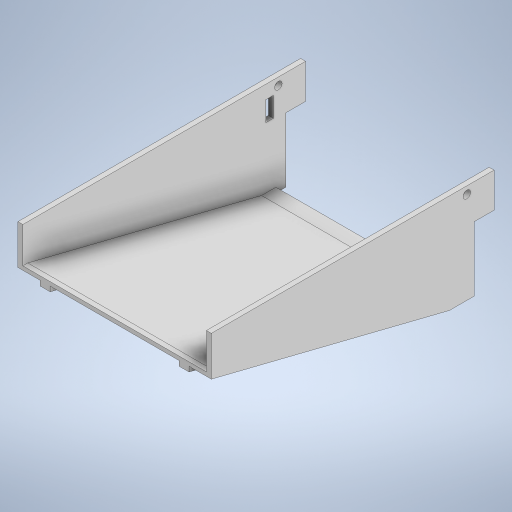
# Autodesk Inventor part: 猫砂盆
Saved by Autodesk Inventor 2023.1 (Build 271208000, 208)
## iProperties
Created: 2023-07-19
Part Number: 猫砂盆
Material: 常规
Document SubType Name: Modeling
Designer: Selcon
Density: 1 g/cm^3
Appearance: 默认
Author: Selcon
Autodesk Inventor part; units mm, degrees
ref_plane "YZ Plane" through (0, 0, 0) normal (1, 0, 0) x (0, 1, 0)
ref_plane "XZ Plane" through (0, 0, 0) normal (0, 1, 0) x (-1, 0, 0)
ref_plane "XY Plane" through (0, 0, 0) normal (0, 0, 1) x (1, 0, 0)
sketch "草图1" plane through (0, 0, 0) normal (0, 0, 1) x (1, 0, 0)
  line L0 (-195, 100) -> (195, 100)
  line L1 (195, 100) -> (195, -100)
  line L2 (195, -100) -> (-195, -100)
  line L3 (-195, -100) -> (-195, 100)
  line L4 (-273, 0) -> (273, 0) projected
  line L5 (0, -140) -> (0, 140) projected
  point P0 (0, 0)
  dimension "d0" = 390
  dimension "d1" = 200
  constraints: 8 end point, 2 parallel, 1 horizontal, 1 perpendicular, 2 other
  measures "d0" distance of L0.start L0.end
  measures "d1" distance of L0.end L1.end
extrude "拉伸1" add sketch "草图1" along normal mid plane 530
sketch "草图2" plane through (195, -100, 265) normal (1, 0, 0) x (0, 0, -1)
  line L0 (0, 200) -> (0, 0) projected
  line L1 (0, 0) -> (0, 120)
  line L2 (0, 120) -> (480, 0)
  line L3 (530, 0) -> (0, 0) projected
  line L4 (480, 0) -> (0, 0)
  point P0 (265, 100)
  dimension "d4" = 120
  dimension "d5" = 480
  constraints: 6 end point, 2 point on line, 1 perpendicular
  measures "d4" distance of L0.end L1.end
  measures "d5" distance of L0.end L2.end
extrude "拉伸2" cut sketch "草图2" against normal through all
shell "抽壳1" thickness 10 removed faces 1 at (-65, 100, 88.3333)
sketch "草图3" plane through (-195, -100, -265) normal (0, -1, 0) x (1, 0, 0)
  line L0 (390, 0) -> (0, 0) projected
  line L1 (10, 0) -> (380, 0)
  line L2 (380, 0) -> (380, 20)
  line L3 (380, 20) -> (10, 20)
  line L4 (10, 20) -> (10, 0)
  line L5 (195, -106) -> (195, 636) projected
  line L6 (0, 0) -> (0, 50) projected
  point P0 (195, 265)
  point P1 (10, 10)
  dimension "d9" = 20
  dimension "d28" = 10
  constraints: 8 end point, 2 parallel, 1 horizontal, 1 midpoint, 1 perpendicular, 1 point on line, 1 other
  measures "d9" distance of L1.end L2.end
  measures "d28" distance between parallel lines of L6 L4
extrude "拉伸3" cut sketch "草图3" against normal through all
sketch "草图4" plane through (195, -100, -265) normal (1, 0, 0) x (0, 0, -1)
  circle A0 centre (-15, 185) radius 7.5
  line L0 (-530, 200) -> (0, 200) projected
  line L1 (0, 200) -> (0, 0) projected
  point P0 (-265, 100)
  dimension "d13" = 15
  dimension "d14" = 15
  dimension "d15" = 15
  constraints: 1 centre point
  measures "d13" distance from line of L0 A0.centre
  measures "d14" diameter of A0
  measures "d15" distance from line of L1 A0.centre
extrude "拉伸4" cut sketch "草图4" against normal through all
sketch "草图5" plane through (-185, -100, -265) normal (1, 0, 0) x (0, 0, -1)
  line L0 (-40, 173) -> (-25, 173)
  line L1 (-25, 173) -> (-25, 133)
  line L2 (-25, 133) -> (-40, 133)
  line L3 (-40, 133) -> (-40, 173)
  circle A0 centre (-15, 185) radius 7.5 projected
  point P0 (-265, 100)
  dimension "d18" = 15
  dimension "d19" = 40
  dimension "d20" = 10
  dimension "d21" = 12
  constraints: 8 end point, 2 parallel, 1 horizontal, 1 perpendicular
  measures "d18" distance of L0.start L0.end
  measures "d19" distance of L0.end L1.end
  measures "d20" distance from line of L1 A0.centre
  measures "d21" distance from line of A0.centre L0
extrude "拉伸5" cut sketch "草图5" against normal through all contours L0 L1 L2 L3
sketch "草图6" plane through (185, 27.8078, 255) normal (0, 0, -1) x (-1, 0, 0)
  line L0 (370, 0) -> (0, 0) projected
  line L1 (370, 72.1922) -> (370, 0) projected
  line L2 (0, 0) -> (370, 0)
  line L3 (370, 0) -> (370, 75)
  line L4 (370, 75) -> (0, 75)
  line L5 (0, 75) -> (0, 0)
  point P0 (185, -27.8078)
  dimension "d24" = 75
  constraints: 8 end point, 2 parallel, 1 horizontal, 1 perpendicular, 1 point on line
  measures "d24" distance of L4.end L0.end
extrude "拉伸6" cut sketch "草图6" against normal through all
sketch "草图10" plane through (-195, -100, -215) normal (0, -0.9701425, 0.2425356) x (1, 0, 0)
  line L0 (0, 494.7727) -> (390, 494.7727) projected
  line L1 (390, 0) -> (0, 0) projected
  line L2 (345, 494.7727) -> (325, 494.7727)
  line L3 (325, 494.7727) -> (325, 0)
  line L4 (325, 0) -> (345, 0)
  line L5 (345, 0) -> (345, 494.7727)
  line L6 (390, 494.7727) -> (390, -48.5071) projected
  point P0 (195, 232.8342)
  point P1 (345, 0)
  dimension "d46" = 20
  dimension "d47" = 45
  constraints: 8 end point, 2 parallel, 2 point on line, 1 horizontal, 1 perpendicular
  measures "d46" distance between parallel lines of L3 L5
  measures "d47" distance between parallel lines of L6 L5
sketch "草图11" plane through (0, 0, 265) normal (0, 0, 1) x (1, 0, 0)
  line L0 (-195, 20) -> (195, 20) projected
  line L1 (150, 20) -> (150, 10)
  line L2 (150, -100) -> (150, 20) projected
  point P0 (0, 0)
  dimension "d50" = 10
  constraints: 2 end point, 1 point on line
  measures "d50" distance of L1.start L1.end
sweep "扫掠1" add profiles "草图10" path "草图11" path curves L1 contours L0 L5 L1 L3
sketch "草图14" plane through (130, -100, -215) normal (-1, 0, 0) x (0, 0.2425356, 0.9701425)
  line L0 (-48.5071, 12.1268) -> (0, 0) projected
  line L1 (0, 0) -> (-2.4254, -9.7014)
  line L2 (-2.4254, -9.7014) -> (36.3803, -19.4029)
  line L3 (36.3803, -19.4029) -> (38.8057, -9.7014)
  line L4 (0, 0) -> (494.7727, 0) projected
  line L5 (38.8057, -9.7014) -> (0, 0)
  line L6 (0, 0) -> (-2.4254, -9.7014) projected
  point P0 (232.8342, 44.8691)
  dimension "d54" = 40
  constraints: 8 end point, 2 equal length, 2 perpendicular, 1 parallel
  measures "d54" distance between parallel lines of L1 L3
extrude "拉伸11" add sketch "草图14" against normal blind 20
sketch "草图15" plane through (0, 0, -265) normal (0, 0, -1) x (-1, 0, 0)
  line L0 (-195, 100) -> (-195, -100) projected
  line L1 (-185, -100) -> (-185, 100) projected
  line L2 (-195, 100) -> (-185, 100)
  line L3 (-185, 100) -> (-185, 30)
  line L4 (-185, 30) -> (-195, 30)
  line L5 (-195, 30) -> (-195, 100)
  point P0 (0, 0)
  point P1 (-195, 30)
  dimension "d57" = 70
  constraints: 8 end point, 2 parallel, 1 horizontal, 1 perpendicular, 1 point on line
  measures "d57" distance between parallel lines of L2 L4
extrude "拉伸12" add sketch "草图15" along normal blind 40
mirror "镜像3" about plane through (0, 0, 0) normal (1, 0, 0) of "扫掠1", "拉伸11"
mirror "镜像4" about plane through (0, 0, 0) normal (1, 0, 0) of "拉伸12"
